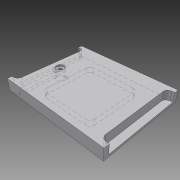
# Autodesk Inventor part: UNLHEP-14-01-P-007_TransportChuck
Saved by Autodesk Inventor 2013 (Build 170138000, 138)
## iProperties
Created: 2014-01-07
Part Number: UNLHEP-14-01-P-007_TransportChuck
Material: Allgemein
Document SubType Name: Modeling
Designer: Frank Meier
Density: 1 g/cm^3
Project: UNL Pixel Phase I
Author: Frank Meier
Revision Number: 00
Autodesk Inventor part; units mm, degrees
ref_plane "YZ Plane" through (0, 0, 0) normal (1, 0, 0) x (0, 1, 0)
ref_plane "XZ Plane" through (0, 0, 0) normal (0, 1, 0) x (-1, 0, 0)
ref_plane "XY Plane" through (0, 0, 0) normal (0, 0, 1) x (1, 0, 0)
sketch "Skizze1" plane through (0, 0, 0) normal (0, 0, 1) x (1, 0, 0)
  line L0 (-115, -90) -> (115, -90)
  line L1 (115, -90) -> (115, 90)
  line L2 (115, 90) -> (-115, 90)
  line L3 (-115, 90) -> (-115, -90)
  line L4 (-115, -90) -> (115, 90) construction
  line L5 (115, -90) -> (-115, 90) construction
  point P0 (0, 0)
  dimension "d0" = 180
  dimension "d2" = 230
  constraints: 12 end point, 2 midpoint, 2 parallel, 1 horizontal, 1 perpendicular
  measures "d0" distance of L0.end L1.end
  measures "d2" distance of L1.end L2.end
extrude "Extrusion1" add sketch "Skizze1" along normal blind 25
ref_plane "Arbeitsebene1" through (-115, 0, 0) normal (0, 1, 0) x (1, 0, 0)
sketch "Skizze2" plane through (-115, 0, 0) normal (0, 1, 0) x (1, 0, 0)
  line L0 (230, 0) -> (230, -25) projected
  line L1 (0, 0) -> (0, -25) projected
  line L2 (230, -25) -> (215, -25)
  line L3 (215, -25) -> (215, -5)
  line L4 (215, -5) -> (230, -5)
  line L5 (230, -5) -> (230, -25)
  line L6 (0, -25) -> (15, -25)
  line L7 (15, -25) -> (15, -5)
  line L8 (15, -5) -> (0, -5)
  line L9 (0, -5) -> (0, -25)
  point P0 (115, 0)
  dimension "d6" = 15
  dimension "d8" = 20
  dimension "d9" = 15
  constraints: 16 end point, 4 parallel, 2 horizontal, 2 perpendicular, 1 collinear
  measures "d6" distance between parallel lines of L5 L3
  measures "d8" distance between parallel lines of L2 L4
  measures "d9" distance between parallel lines of L1 L7
extrude "Extrusion2" cut sketch "Skizze2" along normal mid plane 160
fillet "Rundung1" radius 10 4 edges at (100, 80, 15) (100, -80, 15) (-100, -80, 15) (-100, 80, 15)
sketch "Skizze4" plane through (0, 0, 0) normal (0, 0, -1) x (-1, 0, 0)
  line L0 (-58, -58) -> (58, -58)
  line L1 (58, -58) -> (58, 58)
  line L2 (58, 58) -> (-58, 58)
  line L3 (-58, 58) -> (-58, -58)
  line L4 (-58, -58) -> (58, 58) construction
  line L5 (58, -58) -> (-58, 58) construction
  point P0 (0, 0)
  dimension "d16" = 116
  dimension "d18" = 116
  constraints: 12 end point, 2 midpoint, 2 parallel, 1 horizontal, 1 perpendicular
  measures "d16" distance of L1.end L2.end
  measures "d18" distance of L0.end L1.end
extrude "Extrusion3" cut sketch "Skizze4" against normal blind 12
fillet "Rundung2" radius 10 4 edges at (-58, -58, 6) (58, -58, 6) (58, 58, 6) (-58, 58, 6)
sketch "Skizze7" plane through (0, 0, 25) normal (0, 0, 1) x (1, 0, 0)
  circle A0 centre (-79, 0) radius 10
  line L0 (-100, 70) -> (-100, -70) projected
  point P0 (0, 0)
  dimension "d62" = 20
  dimension "d74" = 21
  constraints: 1 centre point
  measures "d62" diameter of A0
  measures "d74" distance from line of A0.centre L0
extrude "Extrusion6" cut sketch "Skizze7" against normal blind 4
sketch "Skizze8" plane through (0, 0, 0) normal (0, 0, -1) x (-1, 0, 0)
  circle A0 centre (79, 0) radius 10 projected
  point P0 (0, 0)
extrude "Extrusion7" cut sketch "Skizze8" against normal blind 18
sketch "Skizze9" plane through (-79, 0, 18) normal (0, 0, -1) x (-1, 0, 0)
  circle A0 centre (0, 0) radius 10 projected
  circle A1 centre (0, 0) radius 4
  point P0 (-79, 0)
  dimension "d69" = 8
  constraints: 1 centre point, 1 coincident
  measures "d69" diameter of A1
extrude "Extrusion8" cut sketch "Skizze9" against normal blind 5 contours A1
hole "Bohrung4" at (-100, 0, 10) direction (1, 0, 0) diameter 4 depth 50 tip angle 118 counterbore diameter 6 counterbore depth 7
hole "Bohrung5" at (-79, -90, 10) direction (0, 1, 0) diameter 4 depth 90 tip angle 118
